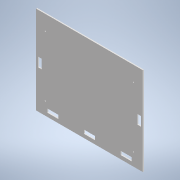
# Autodesk Inventor part: electronic_plate_long_side
Saved by Autodesk Inventor 2021.1 (Build 251245010, 245A)
## iProperties
Created: 2023-01-21
Part Number: electronic_plate_long_side
Material: Типовые
Document SubType Name: Modeling
Designer: zmoze
Density: 1 g/cm^3
Appearance: По умолчанию
Author: zmoze
Autodesk Inventor part; units mm, degrees
ref_plane "YZ Plane" through (0, 0, 0) normal (1, 0, 0) x (0, 1, 0)
ref_plane "XZ Plane" through (0, 0, 0) normal (0, 1, 0) x (-1, 0, 0)
ref_plane "XY Plane" through (0, 0, 0) normal (0, 0, 1) x (1, 0, 0)
sketch "Эскиз1" plane through (0, 0, 0) normal (0, 0, 1) x (1, 0, 0)
  line L0 (-145, 120) -> (145, 120)
  line L1 (145, 120) -> (145, -120)
  line L2 (145, -120) -> (-145, -120)
  line L3 (-145, -120) -> (-145, 120)
  line L4 (-145, 120) -> (145, -120) construction
  line L5 (145, 120) -> (-145, -120) construction
  point P0 (0, 0)
  dimension "d0" = 290
  dimension "d1" = 240
  constraints: 12 end point, 2 midpoint, 2 parallel, 1 horizontal, 1 perpendicular
  measures "d0" distance of L0.start L0.end
  measures "d1" distance of L0.end L1.end
extrude "Выдавливание1" add sketch "Эскиз1" along normal blind 3
sketch "Эскиз2" plane through (0, 0, 3) normal (0, 0, 1) x (1, 0, 0)
  line L0 (-5, 95) -> (5, 95)
  line L1 (145, 120) -> (-145, 120) projected
  line L2 (0, 168) -> (0, -168) projected
  line L3 (-101.423, -89.3301) -> (-106.423, -80.6699)
  line L4 (106.423, -80.6699) -> (101.423, -89.3301)
  point P0 (0, 0)
  point P1 (0, 95)
  point P2 (0, -25)
  point P3 (-103.923, -85)
  point P4 (103.923, -85)
  dimension "d4" = 25
  dimension "d5" = 10
  dimension "d8" = 360
  dimension "d10" = 120
  constraints: 6 end point, 2 point on line, 1 horizontal, 1 midpoint, 13 other
  measures "d4" distance between parallel lines of L0 L1
  measures "d5" distance of L0.start L0.end
  measures "d10" distance from line of point (0, -25) L0
sketch "Эскиз4" plane through (0, 0, 0) normal (0, 0, -1) x (-1, 0, 0)
  line L0 (130, -15.5) -> (130, 9.5) projected
  line L1 (130, 9.5) -> (140, 9.5) projected
  line L2 (140, 9.5) -> (140, -15.5) projected
  line L3 (140, -15.5) -> (130, -15.5) projected
  line L4 (-15, -100) -> (15, -100) projected
  line L5 (15, -100) -> (15, -110) projected
  line L6 (15, -110) -> (-15, -110) projected
  line L7 (-15, -110) -> (-15, -100) projected
  line L8 (115, -100) -> (115, -110) projected
  line L9 (115, -110) -> (85, -110) projected
  line L10 (85, -110) -> (85, -100) projected
  line L11 (85, -100) -> (115, -100) projected
  line L12 (-130, -15.5) -> (-140, -15.5) projected
  line L13 (-140, -15.5) -> (-140, 9.5) projected
  line L14 (-140, 9.5) -> (-130, 9.5) projected
  line L15 (-130, 9.5) -> (-130, -15.5) projected
  circle A0 centre (120, 79) radius 1.5 projected
  circle A1 centre (-120, -85) radius 1.5 projected
  circle A2 centre (120, -85) radius 1.5 projected
  line L16 (-85, -100) -> (-85, -110) projected
  line L17 (-85, -110) -> (-115, -110) projected
  line L18 (-115, -110) -> (-115, -100) projected
  line L19 (-115, -100) -> (-85, -100) projected
  circle A3 centre (-120, 79) radius 1.5 projected
  line L20 (150, 119) -> (-150, 119) projected
  line L21 (-150, 119) -> (-150, -125) projected
  line L22 (-150, -125) -> (150, -125) projected
  line L23 (150, -125) -> (150, 119) projected
  point P0 (0, 0)
extrude "Выдавливание3" cut sketch "Эскиз4" against normal blind 10 contours L0 L1 L2 L3 | L4 L5 L6 L7 | L8 L9 L10 L11 | L12 L13 L14 L15 | A0 | A1 | A2 | L16 L17 L18 L19 | A3
sketch "Эскиз6" plane through (0, 0, 0) normal (0, 0, -1) x (-1, 0, 0)
  circle A0 centre (-115.363, -29) radius 2.5 projected
  circle A1 centre (-115.363, 29) radius 2.5 projected
  circle A2 centre (-74.363, 29) radius 2.5 projected
  circle A3 centre (-74.363, -29) radius 2.5 projected
  circle A4 centre (-25.5005, 12.1735) radius 1.0922 projected
  circle A5 centre (-33.1205, 7.0935) radius 1.0922 projected
  circle A6 centre (-25.5005, 12.1735) radius 1.0922 projected
  circle A7 centre (16.1281, -25.2259) radius 1.5 projected
  circle A8 centre (16.1281, -52.2259) radius 1.5 projected
  circle A9 centre (-13.4032, -52.2259) radius 1.5 projected
  circle A10 centre (-13.4032, -25.2259) radius 1.5 projected
  circle A11 centre (66.1296, 35.3961) radius 1.5875 projected
  circle A12 centre (66.1296, -47.1539) radius 1.5875 projected
  circle A13 centre (114.3896, -40.8039) radius 1.5875 projected
  circle A14 centre (99.1496, -16.6739) radius 1.5875 projected
  circle A15 centre (71.2096, -16.6739) radius 1.5875 projected
  circle A16 centre (114.3896, 34.1261) radius 1.5875 projected
  line L0 (30, 37.5) -> (33, 37.5) projected
  line L1 (30, 34.5) -> (33, 34.5) projected
  line L2 (-33, 37.5) -> (-30, 37.5) projected
  line L3 (-33, 34.5) -> (-30, 34.5) projected
  line L4 (-33, 78.5) -> (-30, 78.5) projected
  line L5 (-33, 81.5) -> (-30, 81.5) projected
  line L6 (30, 78.5) -> (33, 78.5) projected
  line L7 (30, 81.5) -> (33, 81.5) projected
  circle A17 centre (31.5, 36) radius 1.5
  line L8 (33, 34.5) -> (33, 37.5) construction
  line L9 (-30, 34.5) -> (-30, 37.5) construction
  circle A18 centre (-31.5, 36) radius 1.5
  line L10 (33, 78.5) -> (33, 81.5) construction
  circle A19 centre (31.5, 80) radius 1.5
  circle A20 centre (-31.5, 80) radius 1.5
  line L11 (-33, 78.5) -> (-33, 81.5) construction
  point P0 (0, 0)
  dimension "d18" = 3
  constraints: 11 tangent, 8 end point, 4 centre point, 4 vertical, 1 point on line
  measures "d18" diameter of A17
extrude "Выдавливание4" cut sketch "Эскиз6" against normal blind 10
sketch "Эскиз7" plane through (0, 0, 0) normal (0, 0, -1) x (-1, 0, 0)
  circle A0 centre (-95, 80) radius 1.5
  circle A1 centre (95, 80) radius 1.5
  circle A2 centre (95, -80) radius 1.5
  circle A3 centre (-95, -80) radius 1.5
  line L0 (-95, 80) -> (95, 80) construction
  line L1 (95, -80) -> (95, 80) construction
  circle A4 centre (-120, -85) radius 1.5 construction
  line L2 (-95, -80) -> (95, -80) construction
  line L3 (145, -120) -> (-145, -120) construction
  line L4 (-145, 120) -> (145, 120) construction
  line L5 (145, 120) -> (145, -120) construction
  line L6 (-95, 80) -> (-95, -80) construction
  line L7 (-145, -120) -> (-145, 120) construction
  point P0 (0, 0)
  dimension "d19" = 40
  dimension "d20" = 40
  dimension "d21" = 50
  dimension "d22" = 50
  dimension "d23" = 3
  constraints: 8 end point, 4 centre point, 3 equal radius, 2 horizontal, 2 vertical
  measures "d19" distance between parallel lines of L3 L2
  measures "d20" distance between parallel lines of L4 L0
  measures "d21" distance between parallel lines of L5 L1
  measures "d22" distance between parallel lines of L7 L6
  measures "d23" diameter of A1
extrude "Выдавливание5" cut sketch "Эскиз7" against normal blind 10
